Autodesk Inventor part; units mm, degrees
(part 2 of 2)
  line L819 (154.3788, -194.7318) -> (154.3788, -208.7018)
  line L820 (154.3788, -208.7018) -> (153.3983, -208.7018)
  line L821 (149.8982, -208.7018) -> (144.8893, -208.7018)
  line L822 (141.3892, -208.7018) -> (140.4088, -208.7018)
  line L823 (140.4088, -208.7018) -> (140.4088, -194.7318)
  line L824 (140.4088, -194.7318) -> (141.3892, -194.7318)
  line L825 (144.8893, -194.7318) -> (149.8982, -194.7318)
  line L826 (149.8982, -212.969) -> (153.3983, -212.969)
  line L827 (153.3983, -228.5646) -> (149.8982, -228.5646)
  line L828 (144.8893, -228.5646) -> (141.3892, -228.5646)
  line L829 (141.3892, -212.969) -> (144.8893, -212.969)
  line L830 (149.8982, -212.969) -> (149.8982, -213.7818)
  line L831 (149.8982, -227.7518) -> (149.8982, -228.5646)
  line L832 (144.8893, -228.5646) -> (144.8893, -227.7518)
  line L833 (144.8893, -213.7818) -> (144.8893, -212.969)
  line L834 (144.8893, -227.7518) -> (144.8893, -228.5646)
  line L835 (144.8893, -228.5646) -> (141.3892, -228.5646)
  line L836 (141.3892, -228.5646) -> (141.3892, -227.7518)
  line L837 (141.3892, -213.7818) -> (141.3892, -212.969)
  line L838 (141.3892, -212.969) -> (144.8893, -212.969)
  line L839 (144.8893, -212.969) -> (144.8893, -213.7818)
  line L840 (149.8982, -213.7818) -> (149.8982, -212.969)
  line L841 (149.8982, -212.969) -> (153.3983, -212.969)
  line L842 (153.3983, -212.969) -> (153.3983, -213.7818)
  line L843 (153.3983, -227.7518) -> (153.3983, -228.5646)
  line L844 (153.3983, -228.5646) -> (149.8982, -228.5646)
  line L845 (149.8982, -228.5646) -> (149.8982, -227.7518)
  line L846 (153.3983, -213.7818) -> (154.3788, -213.7818)
  line L847 (154.3788, -213.7818) -> (154.3788, -227.7518)
  line L848 (154.3788, -227.7518) -> (153.3983, -227.7518)
  line L849 (149.8982, -227.7518) -> (144.8893, -227.7518)
  line L850 (141.3892, -227.7518) -> (140.4088, -227.7518)
  line L851 (140.4088, -227.7518) -> (140.4088, -213.7818)
  line L852 (140.4088, -213.7818) -> (141.3892, -213.7818)
  line L853 (144.8893, -213.7818) -> (149.8982, -213.7818)
  line L854 (149.8982, -232.019) -> (153.3983, -232.019)
  line L855 (153.3983, -247.6146) -> (149.8982, -247.6146)
  line L856 (144.8893, -247.6146) -> (141.3892, -247.6146)
  line L857 (141.3892, -232.019) -> (144.8893, -232.019)
  line L858 (149.8982, -232.019) -> (149.8982, -232.8318)
  line L859 (149.8982, -246.8018) -> (149.8982, -247.6146)
  line L860 (144.8893, -247.6146) -> (144.8893, -246.8018)
  line L861 (144.8893, -232.8318) -> (144.8893, -232.019)
  line L862 (144.8893, -246.8018) -> (144.8893, -247.6146)
  line L863 (144.8893, -247.6146) -> (141.3892, -247.6146)
  line L864 (141.3892, -247.6146) -> (141.3892, -246.8018)
  line L865 (141.3892, -232.8318) -> (141.3892, -232.019)
  line L866 (141.3892, -232.019) -> (144.8893, -232.019)
  line L867 (144.8893, -232.019) -> (144.8893, -232.8318)
  line L868 (149.8982, -232.8318) -> (149.8982, -232.019)
  line L869 (149.8982, -232.019) -> (153.3983, -232.019)
  line L870 (153.3983, -232.019) -> (153.3983, -232.8318)
  line L871 (153.3983, -246.8018) -> (153.3983, -247.6146)
  line L872 (153.3983, -247.6146) -> (149.8982, -247.6146)
  line L873 (149.8982, -247.6146) -> (149.8982, -246.8018)
  line L874 (153.3983, -232.8318) -> (154.3788, -232.8318)
  line L875 (154.3788, -232.8318) -> (154.3788, -246.8018)
  line L876 (154.3788, -246.8018) -> (153.3983, -246.8018)
  line L877 (149.8982, -246.8018) -> (144.8893, -246.8018)
  line L878 (141.3892, -246.8018) -> (140.4088, -246.8018)
  line L879 (140.4088, -246.8018) -> (140.4088, -232.8318)
  line L880 (140.4088, -232.8318) -> (141.3892, -232.8318)
  line L881 (144.8893, -232.8318) -> (149.8982, -232.8318)
  line L882 (149.8982, -251.069) -> (153.3983, -251.069)
  line L883 (153.3983, -266.6646) -> (149.8982, -266.6646)
  line L884 (144.8893, -266.6646) -> (141.3892, -266.6646)
  line L885 (141.3892, -251.069) -> (144.8893, -251.069)
  line L886 (149.8982, -251.069) -> (149.8982, -251.8818)
  line L887 (149.8982, -265.8518) -> (149.8982, -266.6646)
  line L888 (144.8893, -266.6646) -> (144.8893, -265.8518)
  line L889 (144.8893, -251.8818) -> (144.8893, -251.069)
  line L890 (144.8893, -265.8518) -> (144.8893, -266.6646)
  line L891 (144.8893, -266.6646) -> (141.3892, -266.6646)
  line L892 (141.3892, -266.6646) -> (141.3892, -265.8518)
  line L893 (141.3892, -251.8818) -> (141.3892, -251.069)
  line L894 (141.3892, -251.069) -> (144.8893, -251.069)
  line L895 (144.8893, -251.069) -> (144.8893, -251.8818)
  line L896 (149.8982, -251.8818) -> (149.8982, -251.069)
  line L897 (149.8982, -251.069) -> (153.3983, -251.069)
  line L898 (153.3983, -251.069) -> (153.3983, -251.8818)
  line L899 (153.3983, -265.8518) -> (153.3983, -266.6646)
  line L900 (153.3983, -266.6646) -> (149.8982, -266.6646)
  line L901 (149.8982, -266.6646) -> (149.8982, -265.8518)
  line L902 (153.3983, -251.8818) -> (154.3788, -251.8818)
  line L903 (154.3788, -251.8818) -> (154.3788, -265.8518)
  line L904 (154.3788, -265.8518) -> (153.3983, -265.8518)
  line L905 (149.8982, -265.8518) -> (144.8893, -265.8518)
  line L906 (141.3892, -265.8518) -> (140.4088, -265.8518)
  line L907 (140.4088, -265.8518) -> (140.4088, -251.8818)
  line L908 (140.4088, -251.8818) -> (141.3892, -251.8818)
  line L909 (144.8893, -251.8818) -> (149.8982, -251.8818)
  line L910 (149.8982, -270.119) -> (153.3983, -270.119)
  line L911 (153.3983, -285.7146) -> (149.8982, -285.7146)
  line L912 (144.8893, -285.7146) -> (141.3892, -285.7146)
  line L913 (141.3892, -270.119) -> (144.8893, -270.119)
  line L914 (149.8982, -270.119) -> (149.8982, -270.9318)
  line L915 (149.8982, -284.9018) -> (149.8982, -285.7146)
  line L916 (144.8893, -285.7146) -> (144.8893, -284.9018)
  line L917 (144.8893, -270.9318) -> (144.8893, -270.119)
  line L918 (144.8893, -284.9018) -> (144.8893, -285.7146)
  line L919 (144.8893, -285.7146) -> (141.3892, -285.7146)
  line L920 (141.3892, -285.7146) -> (141.3892, -284.9018)
  line L921 (141.3892, -270.9318) -> (141.3892, -270.119)
  line L922 (141.3892, -270.119) -> (144.8893, -270.119)
  line L923 (144.8893, -270.119) -> (144.8893, -270.9318)
  line L924 (149.8982, -270.9318) -> (149.8982, -270.119)
  line L925 (149.8982, -270.119) -> (153.3983, -270.119)
  line L926 (153.3983, -270.119) -> (153.3983, -270.9318)
  line L927 (153.3983, -284.9018) -> (153.3983, -285.7146)
  line L928 (153.3983, -285.7146) -> (149.8982, -285.7146)
  line L929 (149.8982, -285.7146) -> (149.8982, -284.9018)
  line L930 (153.3983, -270.9318) -> (154.3788, -270.9318)
  line L931 (154.3788, -270.9318) -> (154.3788, -284.9018)
  line L932 (154.3788, -284.9018) -> (153.3983, -284.9018)
  line L933 (149.8982, -284.9018) -> (144.8893, -284.9018)
  line L934 (141.3892, -284.9018) -> (140.4088, -284.9018)
  line L935 (140.4088, -284.9018) -> (140.4088, -270.9318)
  line L936 (140.4088, -270.9318) -> (141.3892, -270.9318)
  line L937 (144.8893, -270.9318) -> (149.8982, -270.9318)
  line L938 (149.8982, -98.669) -> (153.3983, -98.669)
  line L939 (153.3983, -114.2646) -> (149.8982, -114.2646)
  line L940 (144.8893, -114.2646) -> (141.3892, -114.2646)
  line L941 (141.3892, -98.669) -> (144.8893, -98.669)
  line L942 (149.8982, -98.669) -> (149.8982, -99.4818)
  line L943 (149.8982, -113.4518) -> (149.8982, -114.2646)
  line L944 (144.8893, -114.2646) -> (144.8893, -113.4518)
  line L945 (144.8893, -99.4818) -> (144.8893, -98.669)
  line L946 (144.8893, -113.4518) -> (144.8893, -114.2646)
  line L947 (144.8893, -114.2646) -> (141.3892, -114.2646)
  line L948 (141.3892, -114.2646) -> (141.3892, -113.4518)
  line L949 (141.3892, -99.4818) -> (141.3892, -98.669)
  line L950 (141.3892, -98.669) -> (144.8893, -98.669)
  line L951 (144.8893, -98.669) -> (144.8893, -99.4818)
  line L952 (149.8982, -99.4818) -> (149.8982, -98.669)
  line L953 (149.8982, -98.669) -> (153.3983, -98.669)
  line L954 (153.3983, -98.669) -> (153.3983, -99.4818)
  line L955 (153.3983, -113.4518) -> (153.3983, -114.2646)
  line L956 (153.3983, -114.2646) -> (149.8982, -114.2646)
  line L957 (149.8982, -114.2646) -> (149.8982, -113.4518)
  line L958 (153.3983, -99.4818) -> (154.3788, -99.4818)
  line L959 (154.3788, -99.4818) -> (154.3788, -113.4518)
  line L960 (154.3788, -113.4518) -> (153.3983, -113.4518)
  line L961 (149.8982, -113.4518) -> (144.8893, -113.4518)
  line L962 (141.3892, -113.4518) -> (140.4088, -113.4518)
  line L963 (140.4088, -113.4518) -> (140.4088, -99.4818)
  line L964 (140.4088, -99.4818) -> (141.3892, -99.4818)
  line L965 (144.8893, -99.4818) -> (149.8982, -99.4818)
  line L966 (149.8982, -77.2378) -> (153.3983, -77.2378)
  line L967 (153.3983, -92.8334) -> (149.8982, -92.8334)
  line L968 (144.8893, -92.8334) -> (141.3892, -92.8334)
  line L969 (141.3892, -77.2378) -> (144.8893, -77.2378)
  line L970 (149.8982, -77.2378) -> (149.8982, -78.0506)
  line L971 (149.8982, -92.0206) -> (149.8982, -92.8334)
  line L972 (144.8893, -92.8334) -> (144.8893, -92.0206)
  line L973 (144.8893, -78.0506) -> (144.8893, -77.2378)
  line L974 (144.8893, -92.0206) -> (144.8893, -92.8334)
  line L975 (144.8893, -92.8334) -> (141.3892, -92.8334)
  line L976 (141.3892, -92.8334) -> (141.3892, -92.0206)
  line L977 (141.3892, -78.0506) -> (141.3892, -77.2378)
  line L978 (141.3892, -77.2378) -> (144.8893, -77.2378)
  line L979 (144.8893, -77.2378) -> (144.8893, -78.0506)
  line L980 (149.8982, -78.0506) -> (149.8982, -77.2378)
  line L981 (149.8982, -77.2378) -> (153.3983, -77.2378)
  line L982 (153.3983, -77.2378) -> (153.3983, -78.0506)
  line L983 (153.3983, -92.0206) -> (153.3983, -92.8334)
  line L984 (153.3983, -92.8334) -> (149.8982, -92.8334)
  line L985 (149.8982, -92.8334) -> (149.8982, -92.0206)
  line L986 (153.3983, -78.0506) -> (154.3788, -78.0506)
  line L987 (154.3788, -78.0506) -> (154.3788, -92.0206)
  line L988 (154.3788, -92.0206) -> (153.3983, -92.0206)
  line L989 (149.8982, -92.0206) -> (144.8893, -92.0206)
  line L990 (141.3892, -92.0206) -> (140.4088, -92.0206)
  line L991 (140.4088, -92.0206) -> (140.4088, -78.0506)
  line L992 (140.4088, -78.0506) -> (141.3892, -78.0506)
  line L993 (144.8893, -78.0506) -> (149.8982, -78.0506)
  line L994 (168.9482, -289.169) -> (172.4483, -289.169)
  line L995 (172.4483, -304.7646) -> (168.9482, -304.7646)
  line L996 (163.9393, -304.7646) -> (160.4392, -304.7646)
  line L997 (160.4392, -289.169) -> (163.9393, -289.169)
  line L998 (168.9482, -289.169) -> (168.9482, -289.9818)
  line L999 (168.9482, -303.9518) -> (168.9482, -304.7646)
  line L1000 (163.9393, -304.7646) -> (163.9393, -303.9518)
  line L1001 (163.9393, -289.9818) -> (163.9393, -289.169)
  line L1002 (163.9393, -303.9518) -> (163.9393, -304.7646)
  line L1003 (163.9393, -304.7646) -> (160.4392, -304.7646)
  line L1004 (160.4392, -304.7646) -> (160.4392, -303.9518)
  line L1005 (160.4392, -289.9818) -> (160.4392, -289.169)
  line L1006 (160.4392, -289.169) -> (163.9393, -289.169)
  line L1007 (163.9393, -289.169) -> (163.9393, -289.9818)
  line L1008 (168.9482, -289.9818) -> (168.9482, -289.169)
  line L1009 (168.9482, -289.169) -> (172.4483, -289.169)
  line L1010 (172.4483, -289.169) -> (172.4483, -289.9818)
  line L1011 (172.4483, -303.9518) -> (172.4483, -304.7646)
  line L1012 (172.4483, -304.7646) -> (168.9482, -304.7646)
  line L1013 (168.9482, -304.7646) -> (168.9482, -303.9518)
  line L1014 (172.4483, -289.9818) -> (173.4288, -289.9818)
  line L1015 (173.4288, -289.9818) -> (173.4288, -303.9518)
  line L1016 (173.4288, -303.9518) -> (172.4483, -303.9518)
  line L1017 (168.9482, -303.9518) -> (163.9393, -303.9518)
  line L1018 (160.4392, -303.9518) -> (159.4588, -303.9518)
  line L1019 (159.4588, -303.9518) -> (159.4588, -289.9818)
  line L1020 (159.4588, -289.9818) -> (160.4392, -289.9818)
  line L1021 (163.9393, -289.9818) -> (168.9482, -289.9818)
  line L1022 (168.9482, -93.9065) -> (172.4483, -93.9065)
  line L1023 (172.4483, -109.5021) -> (168.9482, -109.5021)
  line L1024 (163.9393, -109.5021) -> (160.4392, -109.5021)
  line L1025 (160.4392, -93.9065) -> (163.9393, -93.9065)
  line L1026 (168.9482, -93.9065) -> (168.9482, -94.7193)
  line L1027 (168.9482, -108.6893) -> (168.9482, -109.5021)
  line L1028 (163.9393, -109.5021) -> (163.9393, -108.6893)
  line L1029 (163.9393, -94.7193) -> (163.9393, -93.9065)
  line L1030 (163.9393, -108.6893) -> (163.9393, -109.5021)
  line L1031 (163.9393, -109.5021) -> (160.4392, -109.5021)
  line L1032 (160.4392, -109.5021) -> (160.4392, -108.6893)
  line L1033 (160.4392, -94.7193) -> (160.4392, -93.9065)
  line L1034 (160.4392, -93.9065) -> (163.9393, -93.9065)
  line L1035 (163.9393, -93.9065) -> (163.9393, -94.7193)
  line L1036 (168.9482, -94.7193) -> (168.9482, -93.9065)
  line L1037 (168.9482, -93.9065) -> (172.4483, -93.9065)
  line L1038 (172.4483, -93.9065) -> (172.4483, -94.7193)
  line L1039 (172.4483, -108.6893) -> (172.4483, -109.5021)
  line L1040 (172.4483, -109.5021) -> (168.9482, -109.5021)
  line L1041 (168.9482, -109.5021) -> (168.9482, -108.6893)
  line L1042 (172.4483, -94.7193) -> (173.4288, -94.7193)
  line L1043 (173.4288, -94.7193) -> (173.4288, -108.6893)
  line L1044 (173.4288, -108.6893) -> (172.4483, -108.6893)
  line L1045 (168.9482, -108.6893) -> (163.9393, -108.6893)
  line L1046 (160.4392, -108.6893) -> (159.4588, -108.6893)
  line L1047 (159.4588, -108.6893) -> (159.4588, -94.7193)
  line L1048 (159.4588, -94.7193) -> (160.4392, -94.7193)
  line L1049 (163.9393, -94.7193) -> (168.9482, -94.7193)
  line L1050 (168.9482, -112.9565) -> (172.4483, -112.9565)
  line L1051 (172.4483, -128.5521) -> (168.9482, -128.5521)
  line L1052 (163.9393, -128.5521) -> (160.4392, -128.5521)
  line L1053 (160.4392, -112.9565) -> (163.9393, -112.9565)
  line L1054 (168.9482, -112.9565) -> (168.9482, -113.7693)
  line L1055 (168.9482, -127.7393) -> (168.9482, -128.5521)
  line L1056 (163.9393, -128.5521) -> (163.9393, -127.7393)
  line L1057 (163.9393, -113.7693) -> (163.9393, -112.9565)
  line L1058 (163.9393, -127.7393) -> (163.9393, -128.5521)
  line L1059 (163.9393, -128.5521) -> (160.4392, -128.5521)
  line L1060 (160.4392, -128.5521) -> (160.4392, -127.7393)
  line L1061 (160.4392, -113.7693) -> (160.4392, -112.9565)
  line L1062 (160.4392, -112.9565) -> (163.9393, -112.9565)
  line L1063 (163.9393, -112.9565) -> (163.9393, -113.7693)
  line L1064 (168.9482, -113.7693) -> (168.9482, -112.9565)
  line L1065 (168.9482, -112.9565) -> (172.4483, -112.9565)
  line L1066 (172.4483, -112.9565) -> (172.4483, -113.7693)
  line L1067 (172.4483, -127.7393) -> (172.4483, -128.5521)
  line L1068 (172.4483, -128.5521) -> (168.9482, -128.5521)
  line L1069 (168.9482, -128.5521) -> (168.9482, -127.7393)
  line L1070 (172.4483, -113.7693) -> (173.4288, -113.7693)
  line L1071 (173.4288, -113.7693) -> (173.4288, -127.7393)
  line L1072 (173.4288, -127.7393) -> (172.4483, -127.7393)
  line L1073 (168.9482, -127.7393) -> (163.9393, -127.7393)
  line L1074 (160.4392, -127.7393) -> (159.4588, -127.7393)
  line L1075 (159.4588, -127.7393) -> (159.4588, -113.7693)
  line L1076 (159.4588, -113.7693) -> (160.4392, -113.7693)
  line L1077 (163.9393, -113.7693) -> (168.9482, -113.7693)
  line L1078 (168.9482, -132.0065) -> (172.4483, -132.0065)
  line L1079 (172.4483, -147.6021) -> (168.9482, -147.6021)
  line L1080 (163.9393, -147.6021) -> (160.4392, -147.6021)
  line L1081 (160.4392, -132.0065) -> (163.9393, -132.0065)
  line L1082 (168.9482, -132.0065) -> (168.9482, -132.8193)
  line L1083 (168.9482, -146.7893) -> (168.9482, -147.6021)
  line L1084 (163.9393, -147.6021) -> (163.9393, -146.7893)
  line L1085 (163.9393, -132.8193) -> (163.9393, -132.0065)
  line L1086 (163.9393, -146.7893) -> (163.9393, -147.6021)
  line L1087 (163.9393, -147.6021) -> (160.4392, -147.6021)
  line L1088 (160.4392, -147.6021) -> (160.4392, -146.7893)
  line L1089 (160.4392, -132.8193) -> (160.4392, -132.0065)
  line L1090 (160.4392, -132.0065) -> (163.9393, -132.0065)
  line L1091 (163.9393, -132.0065) -> (163.9393, -132.8193)
  line L1092 (168.9482, -132.8193) -> (168.9482, -132.0065)
  line L1093 (168.9482, -132.0065) -> (172.4483, -132.0065)
  line L1094 (172.4483, -132.0065) -> (172.4483, -132.8193)
  line L1095 (172.4483, -146.7893) -> (172.4483, -147.6021)
  line L1096 (172.4483, -147.6021) -> (168.9482, -147.6021)
  line L1097 (168.9482, -147.6021) -> (168.9482, -146.7893)
  line L1098 (172.4483, -132.8193) -> (173.4288, -132.8193)
  line L1099 (173.4288, -132.8193) -> (173.4288, -146.7893)
  line L1100 (173.4288, -146.7893) -> (172.4483, -146.7893)
  line L1101 (168.9482, -146.7893) -> (163.9393, -146.7893)
  line L1102 (160.4392, -146.7893) -> (159.4588, -146.7893)
  line L1103 (159.4588, -146.7893) -> (159.4588, -132.8193)
  line L1104 (159.4588, -132.8193) -> (160.4392, -132.8193)
  line L1105 (163.9393, -132.8193) -> (168.9482, -132.8193)
  line L1106 (168.9482, -151.0565) -> (172.4483, -151.0565)
  line L1107 (172.4483, -166.6521) -> (168.9482, -166.6521)
  line L1108 (163.9393, -166.6521) -> (160.4392, -166.6521)
  line L1109 (160.4392, -151.0565) -> (163.9393, -151.0565)
  line L1110 (168.9482, -151.0565) -> (168.9482, -151.8693)
  line L1111 (168.9482, -165.8393) -> (168.9482, -166.6521)
  line L1112 (163.9393, -166.6521) -> (163.9393, -165.8393)
  line L1113 (163.9393, -151.8693) -> (163.9393, -151.0565)
  line L1114 (163.9393, -165.8393) -> (163.9393, -166.6521)
  line L1115 (163.9393, -166.6521) -> (160.4392, -166.6521)
  line L1116 (160.4392, -166.6521) -> (160.4392, -165.8393)
  line L1117 (160.4392, -151.8693) -> (160.4392, -151.0565)
  line L1118 (160.4392, -151.0565) -> (163.9393, -151.0565)
  line L1119 (163.9393, -151.0565) -> (163.9393, -151.8693)
  line L1120 (168.9482, -151.8693) -> (168.9482, -151.0565)
  line L1121 (168.9482, -151.0565) -> (172.4483, -151.0565)
  line L1122 (172.4483, -151.0565) -> (172.4483, -151.8693)
  line L1123 (172.4483, -165.8393) -> (172.4483, -166.6521)
  line L1124 (172.4483, -166.6521) -> (168.9482, -166.6521)
  line L1125 (168.9482, -166.6521) -> (168.9482, -165.8393)
  line L1126 (172.4483, -151.8693) -> (173.4288, -151.8693)
  line L1127 (173.4288, -151.8693) -> (173.4288, -165.8393)
  line L1128 (173.4288, -165.8393) -> (172.4483, -165.8393)
  line L1129 (168.9482, -165.8393) -> (163.9393, -165.8393)
  line L1130 (160.4392, -165.8393) -> (159.4588, -165.8393)
  line L1131 (159.4588, -165.8393) -> (159.4588, -151.8693)
  line L1132 (159.4588, -151.8693) -> (160.4392, -151.8693)
  line L1133 (163.9393, -151.8693) -> (168.9482, -151.8693)
  line L1134 (168.9482, -170.1065) -> (172.4483, -170.1065)
  line L1135 (172.4483, -185.7021) -> (168.9482, -185.7021)
  line L1136 (163.9393, -185.7021) -> (160.4392, -185.7021)
  line L1137 (160.4392, -170.1065) -> (163.9393, -170.1065)
  line L1138 (168.9482, -170.1065) -> (168.9482, -170.9193)
  line L1139 (168.9482, -184.8893) -> (168.9482, -185.7021)
  line L1140 (163.9393, -185.7021) -> (163.9393, -184.8893)
  line L1141 (163.9393, -170.9193) -> (163.9393, -170.1065)
  line L1142 (163.9393, -184.8893) -> (163.9393, -185.7021)
  line L1143 (163.9393, -185.7021) -> (160.4392, -185.7021)
  line L1144 (160.4392, -185.7021) -> (160.4392, -184.8893)
  line L1145 (160.4392, -170.9193) -> (160.4392, -170.1065)
  line L1146 (160.4392, -170.1065) -> (163.9393, -170.1065)
  line L1147 (163.9393, -170.1065) -> (163.9393, -170.9193)
  line L1148 (168.9482, -170.9193) -> (168.9482, -170.1065)
  line L1149 (168.9482, -170.1065) -> (172.4483, -170.1065)
  line L1150 (172.4483, -170.1065) -> (172.4483, -170.9193)
  line L1151 (172.4483, -184.8893) -> (172.4483, -185.7021)
  line L1152 (172.4483, -185.7021) -> (168.9482, -185.7021)
  line L1153 (168.9482, -185.7021) -> (168.9482, -184.8893)
  line L1154 (172.4483, -170.9193) -> (173.4288, -170.9193)
  line L1155 (173.4288, -170.9193) -> (173.4288, -184.8893)
  line L1156 (173.4288, -184.8893) -> (172.4483, -184.8893)
  line L1157 (168.9482, -184.8893) -> (163.9393, -184.8893)
  line L1158 (160.4392, -184.8893) -> (159.4588, -184.8893)
  line L1159 (159.4588, -184.8893) -> (159.4588, -170.9193)
  line L1160 (159.4588, -170.9193) -> (160.4392, -170.9193)
  line L1161 (163.9393, -170.9193) -> (168.9482, -170.9193)
  line L1162 (168.9482, -189.1565) -> (172.4483, -189.1565)
  line L1163 (172.4483, -204.7521) -> (168.9482, -204.7521)
  line L1164 (163.9393, -204.7521) -> (160.4392, -204.7521)
  line L1165 (160.4392, -189.1565) -> (163.9393, -189.1565)
  line L1166 (168.9482, -189.1565) -> (168.9482, -189.9693)
  line L1167 (168.9482, -203.9393) -> (168.9482, -204.7521)
  line L1168 (163.9393, -204.7521) -> (163.9393, -203.9393)
  line L1169 (163.9393, -189.9693) -> (163.9393, -189.1565)
  line L1170 (163.9393, -203.9393) -> (163.9393, -204.7521)
  line L1171 (163.9393, -204.7521) -> (160.4392, -204.7521)
  line L1172 (160.4392, -204.7521) -> (160.4392, -203.9393)
  line L1173 (160.4392, -189.9693) -> (160.4392, -189.1565)
  line L1174 (160.4392, -189.1565) -> (163.9393, -189.1565)
  line L1175 (163.9393, -189.1565) -> (163.9393, -189.9693)
  line L1176 (168.9482, -189.9693) -> (168.9482, -189.1565)
  line L1177 (168.9482, -189.1565) -> (172.4483, -189.1565)
  line L1178 (172.4483, -189.1565) -> (172.4483, -189.9693)
  line L1179 (172.4483, -203.9393) -> (172.4483, -204.7521)
  line L1180 (172.4483, -204.7521) -> (168.9482, -204.7521)
  line L1181 (168.9482, -204.7521) -> (168.9482, -203.9393)
  line L1182 (172.4483, -189.9693) -> (173.4288, -189.9693)
  line L1183 (173.4288, -189.9693) -> (173.4288, -203.9393)
  line L1184 (173.4288, -203.9393) -> (172.4483, -203.9393)
  line L1185 (168.9482, -203.9393) -> (163.9393, -203.9393)
  line L1186 (160.4392, -203.9393) -> (159.4588, -203.9393)
  line L1187 (159.4588, -203.9393) -> (159.4588, -189.9693)
  line L1188 (159.4588, -189.9693) -> (160.4392, -189.9693)
  line L1189 (163.9393, -189.9693) -> (168.9482, -189.9693)
  line L1190 (168.9482, -208.2065) -> (172.4483, -208.2065)
  line L1191 (172.4483, -223.8021) -> (168.9482, -223.8021)
  line L1192 (163.9393, -223.8021) -> (160.4392, -223.8021)
  line L1193 (160.4392, -208.2065) -> (163.9393, -208.2065)
  line L1194 (168.9482, -208.2065) -> (168.9482, -209.0193)
  line L1195 (168.9482, -222.9893) -> (168.9482, -223.8021)
  line L1196 (163.9393, -223.8021) -> (163.9393, -222.9893)
  line L1197 (163.9393, -209.0193) -> (163.9393, -208.2065)
  line L1198 (163.9393, -222.9893) -> (163.9393, -223.8021)
  line L1199 (163.9393, -223.8021) -> (160.4392, -223.8021)
  line L1200 (160.4392, -223.8021) -> (160.4392, -222.9893)
  line L1201 (160.4392, -209.0193) -> (160.4392, -208.2065)
  line L1202 (160.4392, -208.2065) -> (163.9393, -208.2065)
  line L1203 (163.9393, -208.2065) -> (163.9393, -209.0193)
  line L1204 (168.9482, -209.0193) -> (168.9482, -208.2065)
  line L1205 (168.9482, -208.2065) -> (172.4483, -208.2065)
  line L1206 (172.4483, -208.2065) -> (172.4483, -209.0193)
  line L1207 (172.4483, -222.9893) -> (172.4483, -223.8021)
  line L1208 (172.4483, -223.8021) -> (168.9482, -223.8021)
  line L1209 (168.9482, -223.8021) -> (168.9482, -222.9893)
  line L1210 (172.4483, -209.0193) -> (173.4288, -209.0193)
  line L1211 (173.4288, -209.0193) -> (173.4288, -222.9893)
  line L1212 (173.4288, -222.9893) -> (172.4483, -222.9893)
  line L1213 (168.9482, -222.9893) -> (163.9393, -222.9893)
  line L1214 (160.4392, -222.9893) -> (159.4588, -222.9893)
  line L1215 (159.4588, -222.9893) -> (159.4588, -209.0193)
  line L1216 (159.4588, -209.0193) -> (160.4392, -209.0193)
  line L1217 (163.9393, -209.0193) -> (168.9482, -209.0193)
  line L1218 (168.9482, -227.2565) -> (172.4483, -227.2565)
  line L1219 (172.4483, -242.8521) -> (168.9482, -242.8521)
  line L1220 (163.9393, -242.8521) -> (160.4392, -242.8521)
  line L1221 (160.4392, -227.2565) -> (163.9393, -227.2565)
  line L1222 (168.9482, -227.2565) -> (168.9482, -228.0693)
  line L1223 (168.9482, -242.0393) -> (168.9482, -242.8521)
  line L1224 (163.9393, -242.8521) -> (163.9393, -242.0393)
  line L1225 (163.9393, -228.0693) -> (163.9393, -227.2565)
  line L1226 (163.9393, -242.0393) -> (163.9393, -242.8521)
  line L1227 (163.9393, -242.8521) -> (160.4392, -242.8521)
  line L1228 (160.4392, -242.8521) -> (160.4392, -242.0393)
  line L1229 (160.4392, -228.0693) -> (160.4392, -227.2565)
  line L1230 (160.4392, -227.2565) -> (163.9393, -227.2565)
  line L1231 (163.9393, -227.2565) -> (163.9393, -228.0693)
  line L1232 (168.9482, -228.0693) -> (168.9482, -227.2565)
  line L1233 (168.9482, -227.2565) -> (172.4483, -227.2565)
  line L1234 (172.4483, -227.2565) -> (172.4483, -228.0693)
  line L1235 (172.4483, -242.0393) -> (172.4483, -242.8521)
  line L1236 (172.4483, -242.8521) -> (168.9482, -242.8521)
  line L1237 (168.9482, -242.8521) -> (168.9482, -242.0393)
  line L1238 (172.4483, -228.0693) -> (173.4288, -228.0693)
  line L1239 (173.4288, -228.0693) -> (173.4288, -242.0393)
  line L1240 (173.4288, -242.0393) -> (172.4483, -242.0393)
  line L1241 (168.9482, -242.0393) -> (163.9393, -242.0393)
  line L1242 (160.4392, -242.0393) -> (159.4588, -242.0393)
  line L1243 (159.4588, -242.0393) -> (159.4588, -228.0693)
  line L1244 (159.4588, -228.0693) -> (160.4392, -228.0693)
  line L1245 (163.9393, -228.0693) -> (168.9482, -228.0693)
  line L1246 (168.9482, -246.3065) -> (172.4483, -246.3065)
  line L1247 (172.4483, -261.9021) -> (168.9482, -261.9021)
  line L1248 (163.9393, -261.9021) -> (160.4392, -261.9021)
  line L1249 (160.4392, -246.3065) -> (163.9393, -246.3065)
  line L1250 (168.9482, -246.3065) -> (168.9482, -247.1193)
  line L1251 (168.9482, -261.0893) -> (168.9482, -261.9021)
  line L1252 (163.9393, -261.9021) -> (163.9393, -261.0893)
  line L1253 (163.9393, -247.1193) -> (163.9393, -246.3065)
  line L1254 (163.9393, -261.0893) -> (163.9393, -261.9021)
  line L1255 (163.9393, -261.9021) -> (160.4392, -261.9021)
  line L1256 (160.4392, -261.9021) -> (160.4392, -261.0893)
  line L1257 (160.4392, -247.1193) -> (160.4392, -246.3065)
  line L1258 (160.4392, -246.3065) -> (163.9393, -246.3065)
  line L1259 (163.9393, -246.3065) -> (163.9393, -247.1193)
  line L1260 (168.9482, -247.1193) -> (168.9482, -246.3065)
  line L1261 (168.9482, -246.3065) -> (172.4483, -246.3065)
  line L1262 (172.4483, -246.3065) -> (172.4483, -247.1193)
  line L1263 (172.4483, -261.0893) -> (172.4483, -261.9021)
  line L1264 (172.4483, -261.9021) -> (168.9482, -261.9021)
  line L1265 (168.9482, -261.9021) -> (168.9482, -261.0893)
  line L1266 (172.4483, -247.1193) -> (173.4288, -247.1193)
  line L1267 (173.4288, -247.1193) -> (173.4288, -261.0893)
  line L1268 (173.4288, -261.0893) -> (172.4483, -261.0893)
  line L1269 (168.9482, -261.0893) -> (163.9393, -261.0893)
  line L1270 (160.4392, -261.0893) -> (159.4588, -261.0893)
  line L1271 (159.4588, -261.0893) -> (159.4588, -247.1193)
  line L1272 (159.4588, -247.1193) -> (160.4392, -247.1193)
  line L1273 (163.9393, -247.1193) -> (168.9482, -247.1193)
  line L1274 (168.9482, -265.3565) -> (172.4483, -265.3565)
  line L1275 (172.4483, -280.9521) -> (168.9482, -280.9521)
  line L1276 (163.9393, -280.9521) -> (160.4392, -280.9521)
  line L1277 (160.4392, -265.3565) -> (163.9393, -265.3565)
  line L1278 (168.9482, -265.3565) -> (168.9482, -266.1693)
  line L1279 (168.9482, -280.1393) -> (168.9482, -280.9521)
  line L1280 (163.9393, -280.9521) -> (163.9393, -280.1393)
  line L1281 (163.9393, -266.1693) -> (163.9393, -265.3565)
  line L1282 (163.9393, -280.1393) -> (163.9393, -280.9521)
  line L1283 (163.9393, -280.9521) -> (160.4392, -280.9521)
  line L1284 (160.4392, -280.9521) -> (160.4392, -280.1393)
  line L1285 (160.4392, -266.1693) -> (160.4392, -265.3565)
  line L1286 (160.4392, -265.3565) -> (163.9393, -265.3565)
  line L1287 (163.9393, -265.3565) -> (163.9393, -266.1693)
  line L1288 (168.9482, -266.1693) -> (168.9482, -265.3565)
  line L1289 (168.9482, -265.3565) -> (172.4483, -265.3565)
  line L1290 (172.4483, -265.3565) -> (172.4483, -266.1693)
  line L1291 (172.4483, -280.1393) -> (172.4483, -280.9521)
  line L1292 (172.4483, -280.9521) -> (168.9482, -280.9521)
  line L1293 (168.9482, -280.9521) -> (168.9482, -280.1393)
  line L1294 (172.4483, -266.1693) -> (173.4288, -266.1693)
  line L1295 (173.4288, -266.1693) -> (173.4288, -280.1393)
  line L1296 (173.4288, -280.1393) -> (172.4483, -280.1393)
  line L1297 (168.9482, -280.1393) -> (163.9393, -280.1393)
  line L1298 (160.4392, -280.1393) -> (159.4588, -280.1393)
  line L1299 (159.4588, -280.1393) -> (159.4588, -266.1693)
  line L1300 (159.4588, -266.1693) -> (160.4392, -266.1693)
  line L1301 (163.9393, -266.1693) -> (168.9482, -266.1693)
  line L1302 (168.9482, -74.8565) -> (172.4483, -74.8565)
  line L1303 (172.4483, -90.4521) -> (168.9482, -90.4521)
  line L1304 (163.9393, -90.4521) -> (160.4392, -90.4521)
  line L1305 (160.4392, -74.8565) -> (163.9393, -74.8565)
  line L1306 (168.9482, -74.8565) -> (168.9482, -75.6693)
  line L1307 (168.9482, -89.6393) -> (168.9482, -90.4521)
  line L1308 (163.9393, -90.4521) -> (163.9393, -89.6393)
  line L1309 (163.9393, -75.6693) -> (163.9393, -74.8565)
  line L1310 (163.9393, -89.6393) -> (163.9393, -90.4521)
  line L1311 (163.9393, -90.4521) -> (160.4392, -90.4521)
  line L1312 (160.4392, -90.4521) -> (160.4392, -89.6393)
  line L1313 (160.4392, -75.6693) -> (160.4392, -74.8565)
  line L1314 (160.4392, -74.8565) -> (163.9393, -74.8565)
  line L1315 (163.9393, -74.8565) -> (163.9393, -75.6693)
  line L1316 (168.9482, -75.6693) -> (168.9482, -74.8565)
  line L1317 (168.9482, -74.8565) -> (172.4483, -74.8565)
  line L1318 (172.4483, -74.8565) -> (172.4483, -75.6693)
  line L1319 (172.4483, -89.6393) -> (172.4483, -90.4521)
  line L1320 (172.4483, -90.4521) -> (168.9482, -90.4521)
  line L1321 (168.9482, -90.4521) -> (168.9482, -89.6393)
  line L1322 (172.4483, -75.6693) -> (173.4288, -75.6693)
  line L1323 (173.4288, -75.6693) -> (173.4288, -89.6393)
  line L1324 (173.4288, -89.6393) -> (172.4483, -89.6393)
  line L1325 (168.9482, -89.6393) -> (163.9393, -89.6393)
  line L1326 (160.4392, -89.6393) -> (159.4588, -89.6393)
  line L1327 (159.4588, -89.6393) -> (159.4588, -75.6693)
  line L1328 (159.4588, -75.6693) -> (160.4392, -75.6693)
  line L1329 (163.9393, -75.6693) -> (168.9482, -75.6693)
  circle A20 centre (279.9441, -68.3668) radius 3.175
  circle A21 centre (279.9441, -316.0168) radius 3.175
  circle A22 centre (194.2191, -316.0168) radius 3.175
  circle A23 centre (194.2191, -68.3668) radius 3.175
  line L1330 (194.2191, -65.1918) -> (279.9441, -65.1918)
  line L1331 (283.1191, -68.3668) -> (283.1191, -316.0168)
  line L1332 (279.9441, -319.1918) -> (194.2191, -319.1918)
  line L1333 (191.0441, -316.0168) -> (191.0441, -68.3668)
  line L1334 (194.2191, -65.1918) -> (194.2191, -68.3668)
  line L1335 (194.2191, -68.3668) -> (191.0441, -68.3668)
  line L1336 (283.1191, -68.3668) -> (279.9441, -68.3668)
  line L1337 (279.9441, -68.3668) -> (279.9441, -65.1918)
  line L1338 (283.1191, -316.0168) -> (279.9441, -316.0168)
  line L1339 (279.9441, -316.0168) -> (279.9441, -319.1918)
  line L1340 (191.0441, -316.0168) -> (194.2191, -316.0168)
  line L1341 (194.2191, -316.0168) -> (194.2191, -319.1918)
  point P0 (0, 0)
  constraints: 2684 end point, 21 centre point, 16 point on circle, 7 perpendicular, 6 horizontal, 6 tangent, 4 coincident, 4 vertical, 3 horizontal alignment, 1 collinear, 1 concentric, 6 other
extrude "Extrusion1" add sketch "Sketch1" along normal blind 1.5875 contours A0 L1341 L1340 | A0 L1340 A22 L1341 | L1340 L1341 A0 | A0 L1341 A6 L1340 | L1 A23 L0 A20 L3 A21 L2 A22 | L1335 A4 L1334 A23 | A8 L1334 A4 L1335 | L1339 A1 L1338 A7 | A21 L1338 A1 L1339 | L1335 L1334 A4 | A4 L1334 L1335 | L1339 L1338 A1 | A1 L1338 L1339 | L1337 A5 L1336 A20 | A9 L1336 A5 L1337 | L1337 L1336 A5 | A5 L1336 L1337
extrude "Extrusion2" cut sketch "Sketch1" along normal blind 1.5875 contours A0 L1341 L1340 | L1340 L1341 A0 | L1335 L1334 A4 | A4 L1334 L1335 | L1339 L1338 A1 | A1 L1338 L1339 | L1337 L1336 A5 | A5 L1336 L1337
sketch "Sketch6" plane through (0, 1.5875, 0) normal (0, 1, 0) x (1, 0, 0)
  point P0 (0, 0)
body "Solid1"
